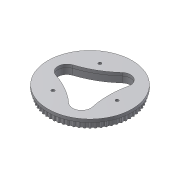
# Autodesk Inventor part: Polea Dentada Grande
Saved by Autodesk Inventor 2020 (Build 240168000, 168)
## iProperties
Part Number: Polea Dentada Grande
Material: Genérico
Document SubType Name: Modeling
Designer: FABLAB
Density: 1 g/cm^3
Appearance: Blanco
Author: FABLAB
Autodesk Inventor part; units mm, degrees
ref_plane "YZ Plane" through (0, 0, 0) normal (1, 0, 0) x (0, 1, 0)
ref_plane "XZ Plane" through (0, 0, 0) normal (0, 1, 0) x (-1, 0, 0)
ref_plane "XY Plane" through (0, 0, 0) normal (0, 0, 1) x (1, 0, 0)
sketch "Boceto1" plane through (0, 0, 0) normal (0, 0, 1) x (1, 0, 0)
  circle A0 centre (26.75, 0) radius 1.5 projected
  arc A1 (20.168, 17.783) -> (20.168, -17.783) centre (101.6471, 0) ccw projected
  arc A2 (5.3165, -26.3575) -> (20.168, -17.783) centre (11.375, -19.7021) ccw projected
  arc A3 (5.3165, -26.3575) -> (-25.4845, -8.5745) centre (-50.8235, -88.0289) ccw projected
  arc A4 (-25.4845, 8.5745) -> (-25.4845, -8.5745) centre (-22.75, 0) ccw projected
  arc A5 (-25.4845, 8.5745) -> (5.3165, 26.3575) centre (-50.8235, 88.0289) ccw projected
  arc A6 (20.168, 17.783) -> (5.3165, 26.3575) centre (11.375, 19.7021) ccw projected
  circle A7 centre (0, 0) radius 42.5 construction
  arc A8 (38.3546, -7.624) -> (-38.3546, -7.624) centre (0, 0) ccw
  circle A9 centre (-13.375, 23.1662) radius 1.5 projected
  circle A10 centre (-13.375, -23.1662) radius 1.5 projected
  circle A11 centre (39.105, 0) radius 1
  line L0 (0, 0) -> (0, -72) construction
  arc A12 (-24.5867, -76.8873) -> (24.5867, -76.8873) centre (0, -72) ccw construction
  line L1 (24.5867, -76.8873) -> (38.3546, -7.624) construction
  line L2 (-24.5867, -76.8873) -> (-38.3546, -7.624) construction
  circle A13 centre (38.9167, 3.833) radius 1
  circle A14 centre (38.3536, 7.629) radius 1
  circle A15 centre (37.4212, 11.3516) radius 1
  circle A16 centre (36.1283, 14.9648) radius 1
  circle A17 centre (34.4875, 18.434) radius 1
  circle A18 centre (32.5146, 21.7256) radius 1
  circle A19 centre (30.2286, 24.8079) radius 1
  circle A20 centre (27.6514, 27.6514) radius 1
  circle A21 centre (24.8079, 30.2286) radius 1
  circle A22 centre (21.7256, 32.5146) radius 1
  circle A23 centre (18.434, 34.4875) radius 1
  circle A24 centre (14.9648, 36.1283) radius 1
  circle A25 centre (11.3516, 37.4212) radius 1
  circle A26 centre (7.629, 38.3536) radius 1
  circle A27 centre (3.833, 38.9167) radius 1
  circle A28 centre (0, 39.105) radius 1
  circle A29 centre (-3.833, 38.9167) radius 1
  circle A30 centre (-7.629, 38.3536) radius 1
  circle A31 centre (-11.3516, 37.4212) radius 1
  circle A32 centre (-14.9648, 36.1283) radius 1
  circle A33 centre (-18.434, 34.4875) radius 1
  circle A34 centre (-21.7256, 32.5146) radius 1
  circle A35 centre (-24.8079, 30.2286) radius 1
  circle A36 centre (-27.6514, 27.6514) radius 1
  circle A37 centre (-30.2286, 24.8079) radius 1
  circle A38 centre (-32.5146, 21.7256) radius 1
  circle A39 centre (-34.4875, 18.434) radius 1
  circle A40 centre (-36.1283, 14.9648) radius 1
  circle A41 centre (-37.4212, 11.3516) radius 1
  circle A42 centre (-38.3536, 7.629) radius 1
  circle A43 centre (-38.9167, 3.833) radius 1
  circle A44 centre (-39.105, 0) radius 1
  circle A45 centre (-38.9167, -3.833) radius 1
  circle A46 centre (-38.3536, -7.629) radius 1
  circle A47 centre (-37.4212, -11.3516) radius 1
  circle A48 centre (-36.1283, -14.9648) radius 1
  circle A49 centre (-34.4875, -18.434) radius 1
  circle A50 centre (-32.5146, -21.7256) radius 1
  circle A51 centre (-30.2286, -24.8079) radius 1
  circle A52 centre (-27.6514, -27.6514) radius 1
  circle A53 centre (-24.8079, -30.2286) radius 1
  circle A54 centre (-21.7256, -32.5146) radius 1
  circle A55 centre (-18.434, -34.4875) radius 1
  circle A56 centre (-14.9648, -36.1283) radius 1
  circle A57 centre (-11.3516, -37.4212) radius 1
  circle A58 centre (-7.629, -38.3536) radius 1
  circle A59 centre (-3.833, -38.9167) radius 1
  circle A60 centre (0, -39.105) radius 1
  circle A61 centre (3.833, -38.9167) radius 1
  circle A62 centre (7.629, -38.3536) radius 1
  circle A63 centre (11.3516, -37.4212) radius 1
  circle A64 centre (14.9648, -36.1283) radius 1
  circle A65 centre (18.434, -34.4875) radius 1
  circle A66 centre (21.7256, -32.5146) radius 1
  circle A67 centre (24.8079, -30.2286) radius 1
  circle A68 centre (27.6514, -27.6514) radius 1
  circle A69 centre (30.2286, -24.8079) radius 1
  circle A70 centre (32.5146, -21.7256) radius 1
  circle A71 centre (34.4875, -18.434) radius 1
  circle A72 centre (36.1283, -14.9648) radius 1
  circle A73 centre (37.4212, -11.3516) radius 1
  circle A74 centre (38.3536, -7.629) radius 1
  arc A75 (-38.3546, -7.624) -> (38.3546, -7.624) centre (0, 0) ccw construction
  circle A76 centre (0, 0) radius 39.105
  circle A77 centre (38.9167, -3.833) radius 1
  point P0 (0, 0)
  dimension "d0" = 78.21
  dimension "d9" = 2
  dimension "d11" = 72
  dimension "d20" = 68.565
  dimension "d21" = 138.1983
  dimension "d22" = 70.6184
  dimension "d23" = 25.0677
  dimension "d26" = 360
  dimension "d28" = 3.8376
  constraints: 67 centre point, 7 point on circle, 6 end point, 6 tangent, 3 coincident, 1 horizontal alignment, 1 vertical, 132 other
  measures "d0" diameter of A8
  measures "d9" diameter of A11
  measures "d11" distance of L0.start L0.end
  measures "d22" distance of L1.start L1.end
  measures "d23" radius of A12
  measures "d28" distance of A19.centre A20.centre
extrude "Extrusión1" add sketch "Boceto1" along normal blind 6
sketch "Boceto2" plane through (0, 0, 6) normal (0, 0, 1) x (1, 0, 0)
  circle A0 centre (0, 0) radius 41.5
  arc A1 (20.168, 17.783) -> (20.168, -17.783) centre (101.6471, 0) ccw
  arc A2 (20.168, 17.783) -> (5.3165, 26.3575) centre (11.375, 19.7021) ccw projected
  arc A3 (-25.4845, 8.5745) -> (5.3165, 26.3575) centre (-50.8235, 88.0289) ccw
  arc A4 (-25.4845, 8.5745) -> (-25.4845, -8.5745) centre (-22.75, 0) ccw
  arc A5 (5.3165, -26.3575) -> (-25.4845, -8.5745) centre (-50.8235, -88.0289) ccw projected
  arc A6 (5.3165, -26.3575) -> (20.168, -17.783) centre (11.375, -19.7021) ccw projected
  circle A7 centre (-13.375, -23.1662) radius 1.5 projected
  circle A8 centre (-13.375, 23.1662) radius 1.5 projected
  circle A9 centre (26.75, 0) radius 1.5 projected
  dimension "d30" = 83
  constraints: 6 point on circle, 4 centre point, 1 coincident, 11 other
  measures "d30" diameter of A0
extrude "Extrusión2" add sketch "Boceto2" along normal blind 3 separate body
sketch "Boceto3" plane through (0, 0, 0) normal (0, 0, -1) x (-1, 0, 0)
  circle A0 centre (0, 0) radius 41.5 projected
  circle A1 centre (0, 0) radius 36
  point P0 (0, 0)
  dimension "d6" = 5.5
  constraints: 1 centre point
  measures "d6" radial gap between concentric circles of A0 A1
